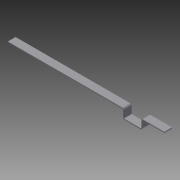
# Autodesk Inventor part: Cylinder Mount
Saved by Autodesk Inventor 2013 (Build 170138000, 138)
## iProperties
Created: 2013-01-26
Part Number: Cylinder Mount
Material: Generic
Document SubType Name: Sheet Metal
Designer: actoennies
Density: 1 g/cm^3
Sheet Metal Rule: Default
Author: actoennies
Autodesk Inventor part; units mm, degrees
ref_plane "YZ Plane" through (0, 0, 0) normal (1, 0, 0) x (0, 1, 0)
ref_plane "XZ Plane" through (0, 0, 0) normal (0, 1, 0) x (-1, 0, 0)
ref_plane "XY Plane" through (0, 0, 0) normal (0, 0, 1) x (1, 0, 0)
sketch "Sketch1" plane through (0, 0, 0) normal (0, 1, 0) x (-1, 0, 0)
  line L0 (0, 0) -> (0, 25.4)
  line L1 (0, 25.4) -> (50.8, 25.4)
  line L2 (50.8, 25.4) -> (50.8, 0)
  line L3 (50.8, 0) -> (0, 0)
  dimension "d0" = 25.4
  dimension "d1" = 50.8
  measures "d0" distance of L0.start L0.end
  measures "d1" distance of L0.end L1.end
extrude "Plate1" add sketch "Sketch1" along normal blind 3.175
sketch "Sketch2" plane through (3.175, 6.35, 0) normal (1, 0, 0) x (0, 1, 0)
  line L0 (0, 25.4) -> (0, 0)
  line L1 (0, 0) -> (19.05, 0)
  line L2 (19.05, 0) -> (19.05, 25.4)
  line L3 (19.05, 25.4) -> (0, 25.4)
  constraints: 6 end point, 1 horizontal, 1 perpendicular, 1 vertical
edge flange "Flange1" height 25.4 angle 90 thickness 3.175 bend radius 3.175 thickness toward (1, 0, 0) relief straight relief width 3.175 relief depth 1.5875 corner gap 3.175 corner form 0 edges at (0, 3.175, 12.7) (-50.8, 3.175, 12.7) wall of the first edge with corners at (3.175, 6.35, 25.4) (3.175, 6.35, 0) (3.175, 25.4, 0) (3.175, 25.4, 25.4)
bend "Bend1"
corner "Corner1"
sketch "Sketch3" plane through (9.525, 28.575, 25.4) normal (0, 1, 0) x (-1, 0, 0)
  line L0 (0, -25.4) -> (0, 0)
  line L1 (0, 0) -> (-69.85, 0)
  line L2 (-69.85, 0) -> (-69.85, -25.4)
  line L3 (-69.85, -25.4) -> (0, -25.4)
  constraints: 6 end point, 1 horizontal, 1 perpendicular, 1 vertical
edge flange "Flange2" height 76.2 angle 90 thickness 3.175 bend radius 3.175 thickness toward (0, 1, 0) relief straight relief width 3.175 relief depth 1.5875 edges at (6.35, 25.4, 12.7) wall of the first edge with corners at (9.525, 28.575, 0) (9.525, 28.575, 25.4) (79.375, 28.575, 25.4) (79.375, 28.575, 0)
bend "Bend2"
corner "Corner2"
sketch "Sketch4" plane through (-60.325, 28.575, 0) normal (0, 1, 0) x (-1, 0, 0)
  line L0 (0, 25.4) -> (0, 0)
  line L1 (0, 0) -> (374.65, 0)
  line L2 (374.65, 0) -> (374.65, 25.4)
  line L3 (374.65, 25.4) -> (0, 25.4)
  constraints: 6 end point, 1 horizontal, 1 perpendicular, 1 vertical
edge flange "Flange3" height 381 angle 90 thickness 3.175 bend radius 3.175 thickness toward (0, 1, 0) relief straight relief width 3.175 relief depth 1.5875 edges at (-57.15, 25.4, 12.7) wall of the first edge with corners at (-60.325, 28.575, 25.4) (-60.325, 28.575, 0) (-434.975, 28.575, 0) (-434.975, 28.575, 25.4)
bend "Bend3"
corner "Corner3"
equation "\"d3\" = BendReliefWidth"
equation "\"d4\" = BendReliefDepth"
equation "\"d5\" = MinimumRemnant"
equation "\"d6\" = BendRadius"
equation "\"d9\" = BendRadius"
equation "\"d10\" = CornerReliefSize"
equation "\"d11\" = GapSize"
equation "\"d12\" = JacobiRadiusSize"
equation "\"d13\" = BendReliefWidth"
equation "\"d14\" = BendReliefDepth"
equation "\"d15\" = MinimumRemnant"
equation "\"d16\" = BendRadius"
equation "\"d19\" = BendRadius"
equation "\"d20\" = CornerReliefSize"
equation "\"d21\" = GapSize"
equation "\"d22\" = JacobiRadiusSize"
equation "\"d23\" = BendReliefWidth"
equation "\"d24\" = BendReliefDepth"
equation "\"d25\" = MinimumRemnant"
equation "\"d26\" = BendRadius"
equation "\"d29\" = BendRadius"
equation "\"d30\" = CornerReliefSize"
equation "\"d31\" = GapSize"
equation "\"d32\" = JacobiRadiusSize"
equation "\"BendRadius\" = Thickness"
equation "\"BendReliefWidth\" = Thickness"
equation "\"BendReliefDepth\" = 0.5 * Thickness"
equation "\"CornerReliefSize\" = 4 * Thickness"
equation "\"MinimumRemnant\" = 2 * Thickness"
equation "\"TransitionRadius\" = BendRadius"
equation "\"JacobiRadiusSize\" = BendRadius"
equation "\"GapSize\" = Thickness"
equation "\"d2\" = BendRadius"
equation "\"Thickness\" = 3.175"
body "Solid1"
